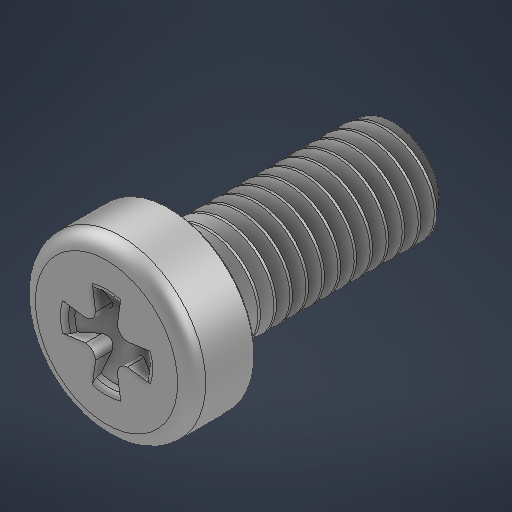
# Autodesk Inventor part: M5x14L_Hex
Saved by Autodesk Inventor 2025.2 (Build 292293000, 293)
## iProperties
Created: 2024-12-01
Part Number: M5x14L_Hex
Material: Generic
Document SubType Name: Modeling
Designer: Tiago
Density: 1 g/cm^3
Appearance: Anodized - Light Gray
Author: Tiago
Autodesk Inventor part; units mm, degrees
ref_plane "YZ Plane" through (0, 0, 0) normal (1, 0, 0) x (0, 1, 0)
ref_plane "XZ Plane" through (0, 0, 0) normal (0, 1, 0) x (-1, 0, 0)
sketch "Sketch2" plane through (0, 0, 0) normal (0, 1, 0) x (-1, 0, 0)
  line L0 (0, -1.5) -> (0, -14.6)
  line L1 (-1.8865, -14.6) -> (-1.8865, -3.2)
  line L2 (-4.25, 0) -> (-2.125, 0)
  line L3 (-1.9507, -0.3738) -> (0, -1.5)
  line L4 (-2.125, 0) -> (-1.9507, -0.3738)
  line L5 (-4.25, 0) -> (-4.25, -3.2)
  line L6 (-4.25, -3.2) -> (-1.8865, -3.2)
  line L7 (-1.8865, -14.6) -> (0, -14.6)
  line L8 (0, -14.6) -> (-2.5, -14.6)
  line L9 (-2.5, -14.6) -> (-2.5, -16.6)
  line L10 (-2.5, -16.6) -> (0, -16.6)
  line L11 (0, -16.6) -> (0, -14.6)
  line L12 (-2.5, -14.6) -> (-2.5, -11.1)
  line L13 (-1.8865, -14.6) -> (-2.5, -14.2458)
  point P0 (0, 0)
  point P1 (-3.1875, 0)
  point P2 (0, -11.7)
  point P3 (-2.5, -12.508)
  point P4 (-1.8865, -14.6)
  dimension "d0" = 3.773
  dimension "d3" = 4.25
  dimension "d4" = 60
  dimension "d5" = 25
  dimension "d6" = 1.5
  dimension "k" = 3.2
  dimension "L" = 14.6
  dimension "d79" = 8.5
  dimension "d84" = 5
  dimension "d91" = 30
  dimension "d92" = 2
  dimension "d93" = 2
  constraints: 28 end point, 5 point on line, 3 parallel, 3 vertical, 2 horizontal, 2 horizontal alignment, 2 perpendicular, 1 midpoint
  measures "d0" diameter of L1 L0
  measures "d3" diameter of L2.end L0
  measures "d4" angle of L3 L0
  measures "d5" angle of L0 L4
  measures "d6" vertical distance of L0.start point (-3.188, 0)
  measures "k" vertical distance of L1.end L2.start
  measures "L" distance from line of L0.end L2
  measures "d79" diameter of L2.start L0
  measures "d84" diameter of L9 L0
  measures "d91" angle of L8 L13
  measures "d92" distance between parallel lines of L7 L10
  measures "d93" distance between parallel lines of L10 L8
revolve "Revolution1" add sketch "Sketch2" angle 360 about axis through (0, 0, -1.5) along (0, 0, -1) contours L0 L7 L1 L6 L5 L2 L4 L3
sketch "Sketch3" plane through (0, 0, 0) normal (0, 0, 1) x (1, 0, 0)
  line L0 (0, 5.95) -> (0, -5.95) projected
  line L1 (-5.95, 0) -> (5.95, 0) projected
  circle A0 centre (0, 0) radius 2.125 projected
  line L2 (0, 2.125) -> (0.6965, 2.125) construction
  line L3 (0, 2.125) -> (-0.697, 2.125)
  line L4 (2.125, 0) -> (2.125, 0.6965) construction
  line L5 (2.125, 0) -> (2.125, -0.6965) construction
  line L6 (-0.697, 2.125) -> (-0.697, 2.0074)
  line L7 (0.6965, 2.125) -> (0.6965, 2.0076)
  line L8 (2.0076, 0.6965) -> (2.125, 0.6965)
  arc A1 (2.125, 0.6965) -> (0.6965, 2.125) centre (0, 0) ccw
  line L9 (-0.697, -0.2035) -> (-0.697, 0.1455) construction
  line L10 (-0.5455, 1.0455) -> (0.5455, 1.0455) construction
  line L11 (-0.697, 2.125) -> (-0.5455, 1.0455)
  line L12 (0.6965, 2.125) -> (0.5455, 1.0455)
  line L13 (0.6965, 0.6965) -> (1.0455, 0.6965) construction
  line L14 (1.0455, -0.5455) -> (1.0455, 0.5455) construction
  line L15 (1.0455, 0.5455) -> (2.125, 0.6965)
  line L16 (1.0455, -0.5455) -> (2.125, -0.6965)
  line L17 (0.6965, 0.6965) -> (0.6965, 1.0455) construction
  arc A2 (0.5455, 1.0455) -> (1.0455, 0.5455) centre (1.0617, 1.0617) ccw
  line L18 (-2.125, 0) -> (-2.125, 0.6965) construction
  arc A3 (-0.6965, 2.125) -> (-2.125, 0.6965) centre (0, 0) ccw
  line L19 (-1.0455, 0.5455) -> (-2.125, 0.6965)
  arc A4 (-1.0455, 0.5455) -> (-0.5455, 1.0455) centre (-1.0617, 1.0617) ccw
  line L20 (0, -2.125) -> (0.6965, -2.125) construction
  line L21 (0, -2.125) -> (-0.697, -2.125) construction
  line L22 (-0.697, -2.125) -> (-0.5455, -1.0455)
  line L23 (0.6965, -2.125) -> (0.5455, -1.0455)
  arc A5 (1.0455, -0.5455) -> (0.5455, -1.0455) centre (1.0617, -1.0617) ccw
  arc A6 (-0.5455, -1.0455) -> (-1.0455, -0.5455) centre (-1.0617, -1.0617) ccw
  line L24 (-2.125, 0) -> (-2.125, -0.6965) construction
  line L25 (-1.0455, -0.5455) -> (-2.125, -0.6965)
  arc A7 (-2.125, -0.6965) -> (-0.697, -2.125) centre (0.6652, 0.6647) ccw
  arc A8 (0.6965, -2.125) -> (3.6906, -0.032) centre (0.7558, 0.9781) ccw
  point P0 (0, 0)
  point P1 (0, 1.0455)
  point P2 (1.0455, 0)
  point P3 (-2.013, -0.6808)
  point P4 (-0.6813, -2.0128)
  point P5 (-0.6813, 2.0128)
  point P6 (-2.013, 0.6808)
  point P7 (0.6808, -2.013)
  point P8 (2.013, -0.6808)
  point P9 (2.013, 0.6808)
  point P10 (0.6808, 2.013)
  dimension "d12" = 0.6965
  dimension "d13" = 0.697
  dimension "d14" = 0.6965
  dimension "d15" = 0.6965
  dimension "d17" = 0.349
  dimension "d20" = 1.091
  dimension "d21" = 0.349
  dimension "d22" = 1.091
  constraints: 48 end point, 23 point on circle, 14 symmetric about line, 8 centre point, 6 point on line, 4 horizontal, 4 vertical, 2 midpoint, 2 perpendicular, 2 tangent, 4 other
  measures "d12" distance of L2.start L2.end
  measures "d13" distance of L2.start L3.end
  measures "d14" distance of L4.start L4.end
  measures "d15" distance of L4.start L5.end
  measures "d17" distance of L9.start L9.end
  measures "d20" distance of L10.start L10.end
  measures "d21" distance of L13.start L13.end
  measures "d22" distance of L14.start L14.end
extrude "Extrusion1" add sketch "Sketch3" against normal up to next contours A0 L15 A2 L12 | L11 A4 L19 A0 | A0 L25 A6 L22 | L23 A5 L16 A0
fillet "Fillet1" radius 0.274 4 edges at (-0.0002, 2.125, 0) (2.125, 0, 0) (-0.0002, -2.125, 0) (-2.125, 0, 0)
sketch "Sketch4" plane through (0, 0, 0) normal (0, 1, 0) x (-1, 0, 0)
  line L0 (0, -19.1273) -> (0, 3.2301) projected
  line L1 (-2.5, -15.4542) -> (-2.5, -15.5792)
  line L2 (-2.5, -15.5792) -> (-1.8865, -15.9334)
  line L3 (-1.8865, -15.9334) -> (-1.8865, -15.1)
  line L4 (-2.5, -15.4542) -> (-1.8865, -15.1)
  line L5 (-2.5, -15.5167) -> (-1.8865, -15.5167)
  line L6 (0, -10) -> (0, -9)
  line L7 (2.1429, -9) -> (-2.1429, -9)
  line L8 (-1.8865, -3.2) -> (-4.25, -3.2) projected
  line L9 (-4.25, -3.2) -> (-4.25, 0) projected
  line L10 (4.25, 0) -> (4.25, -3.2) projected
  line L11 (4.25, -3.2) -> (1.8865, -3.2) projected
  line L12 (-4.25, 0) -> (-2.2996, 0) projected
  line L13 (-1.9507, -0.3738) -> (0, -1.5) projected
  line L14 (0, -1.5) -> (1.9507, -0.3738) projected
  line L15 (2.2996, 0) -> (4.25, 0) projected
  line L16 (1.8865, -3.2) -> (1.8865, -14.6) projected
  line L17 (-1.8865, -14.6) -> (-1.8865, -3.2) projected
  line L18 (1.8865, -14.6) -> (-1.8865, -14.6) projected
  line L19 (1.9507, -0.3738) -> (2.0512, -0.1582) projected
  arc A0 (2.2996, 0) -> (2.0512, -0.1582) centre (2.2996, -0.274) ccw projected
  arc A1 (-2.0512, -0.1582) -> (-2.2996, 0) centre (-2.2996, -0.274) ccw projected
  line L20 (-2.0512, -0.1582) -> (-1.9507, -0.3738) projected
  point P0 (0, 0)
  point P1 (-2.5, -14.9542)
  point P2 (0, -10.9667)
  dimension "d" = 3.773
  dimension "d28" = 0.5
  dimension "d77" = 0.125
  dimension "d78" = 60
  dimension "d81" = 0.5
  dimension "d90" = 0.6135
  constraints: 14 end point, 3 midpoint, 3 point on line, 2 horizontal, 1 equal length, 1 parallel, 1 vertical
  measures "d" diameter of L3 L0
  measures "d28" distance of point (-2.5, -14.954) L1.start
  measures "d77" distance of L1.start L1.end
  measures "d78" angle of L2 L4
  measures "d81" distance of L17.start L3.end
  measures "d90" distance of L5.start L5.end
coil "Coil1" sketch "Sketch4" operation add axis through (0, 0, -10) along (0, 0, 1) pitch 0.8 turns 15.75 hand right contours L4 L3 L5 L1 | L5 L3 L2 L1
ref_plane "Work Plane1" through (0, 0, -3) normal (0, 0, 1) x (1, 0, 0)
chamfer "Chamfer5" distance 0.1 angle 45 1 edges at (-4.25, 0, -3.2)
fillet "Fillet3" radius 0.7 1 edges at (-4.25, 0, 0)
revolve "Revolution3" cut sketch "Sketch2" angle 360 about axis through (0, 0, -1.5) along (0, 0, -1) contours L11 L10 L9 L8 L7 | L8 L12 L13
equation "\"M\" = 5"
body "Solid1"
